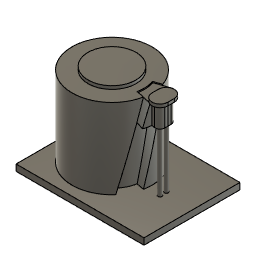
CAM+loft (Autodesk Fusion 360 design; units mm, degrees)
Autodesk Fusion 360 part; units mm, degrees
cylinder "CylinderPrimitive1" add diameter 25 height 25 placed x (1, 0, 0) y (0, 0, -1) z (0, 1, 0) at (0, 0, 0) makes body 1 in component "CAM"
ref_plane "WorkPlane1" through (0, 12.5, 0) normal (0, 1, 0) x (1, 0, 0)
ref_plane "WorkPlane2" through (0, 6.25, 0) normal (0, 1, 0) x (0, 0, 1)
ref_plane "WorkPlane3" through (0, 18.75, 0) normal (0, 1, 0) x (1, 0, 0)
sketch "Sketch2" plane through (0, 0, 0) normal (0, -1, 0) x (1, 0, 0)
  circle A0 centre (0, 0) radius 12.5
  line L0 (10, 0) -> (15, 0)
  line L1 (8.6603, 5) -> (12.9904, 7.5)
  arc A1 (15, 0) -> (12.9904, 7.5) centre (0, 0) ccw
  arc A2 (10, 0) -> (8.6603, 5) centre (0, 0) ccw
  line L2 (8.6603, 5) -> (0, 0) construction
  line L3 (0, 0) -> (10, 0) construction
  line L4 (0, 0) -> (14.4889, 3.8823) construction
  line L5 (9.6593, 2.5882) -> (14.4889, 3.8823) construction
  point P0 (12.0741, 3.2352)
  dimension "d3" = 30
  dimension "d4" = 30
  dimension "d5" = 20
  constraint horizontal L0
  constraint coincident A0.centre A1.centre
  constraint parallel L1 L2
  constraint parallel L0 L3
  constraint midpoint A1 L4.end
  constraint midpoint A2 L5.start
  constraint midpoint L5 P0
  measures "d3" diameter of A1
  measures "d4" angle of L0 L1
  measures "d5" diameter of A2
sketch "Sketch3" plane through (0, 6.25, 0) normal (0, 1, 0) x (1, 0, 0)
  circle A0 centre (0, 0) radius 12.5 construction
  line L0 (9.2388, -3.8268) -> (13.8582, -5.7403)
  line L1 (9.9144, 1.3053) -> (14.8717, 1.9579)
  line L2 (0, 0) -> (15, 0) construction
  line L3 (10, 0) -> (15, 0) construction
  arc A1 (9.2388, -3.8268) -> (9.9144, 1.3053) centre (0, 0) ccw
  arc A2 (13.8582, -5.7403) -> (14.8717, 1.9579) centre (0, 0) ccw
  line L4 (9.2388, -3.8268) -> (0, 0) construction
  line L5 (9.9144, 1.3053) -> (0, 0) construction
  line L6 (0, 0) -> (14.8717, -1.9579) construction
  line L7 (14.8717, -1.9579) -> (9.9144, -1.3053) construction
  point P0 (12.3931, -1.6316)
  dimension "d6" = 30
  dimension "d7" = 20
  dimension "d8" = 30
  dimension "d9" = 7.5
  constraint concentric A0 A2
  constraint concentric A0 A1
  constraint coincident A0.centre L2.start
  constraint coincident L2.end A2
  constraint horizontal L2
  constraint parallel L0 L4
  constraint midpoint A2 L6.end
  constraint midpoint A1 L7.end
  constraint parallel L6 L7
  constraint midpoint L7 P0
  measures "d6" diameter of A2
  measures "d7" diameter of A1
  measures "d8" angle of L0 L1
  measures "d9" angle of L1 L3
sketch "Sketch4" plane through (0, 12.5, 0) normal (0, 1, 0) x (1, 0, 0)
  line L0 (9.6593, -2.5882) -> (14.4889, -3.8823) construction
  line L1 (0, 0) -> (15, 0) construction
  line L2 (9.6593, 2.5882) -> (14.4889, 3.8823)
  line L3 (0, 0) -> (14.4889, -3.8823) construction
  line L4 (10, 0) -> (15, 0) construction
  arc A0 (9.6593, -2.5882) -> (9.6593, 2.5882) centre (0, 0) ccw
  arc A1 (14.4889, -3.8823) -> (14.4889, 3.8823) centre (0, 0) ccw
  line L5 (14.4889, -3.8823) -> (9.6593, -2.5882)
  line L6 (9.6593, 2.5882) -> (0, 0) construction
  point P0 (12.5, 0)
  dimension "d10" = 30
  dimension "d11" = 20
  dimension "d13" = 30
  dimension "d14" = 15
  dimension "d15" = 30
  constraint coincident L1.start L3.start
  constraint concentric A0 A1
  constraint coincident L1.end A1
  constraint horizontal L1
  constraint coincident L0.end L3.end
  constraint parallel L3 L5
  constraint midpoint L4 P0
  measures "d10" diameter of A1
  measures "d11" diameter of A0
  measures "d13" angle of L0 L2
  measures "d14" angle of L2 L4
  measures "d15" angle of L3 L6
sketch "Sketch5" plane through (0, 18.75, 0) normal (0, 1, 0) x (1, 0, 0)
  line L0 (0, 0) -> (13.8582, 5.7403)
  line L1 (10, 0) -> (15, 0) construction
  arc A0 (14.8717, -1.9579) -> (13.8582, 5.7403) centre (0, 0) ccw
  arc A1 (9.9144, -1.3053) -> (9.2388, 3.8268) centre (0, 0) ccw
  line L2 (14.8717, -1.9579) -> (9.9144, -1.3053)
  line L3 (9.9144, -1.3053) -> (0, 0) construction
  line L4 (9.9144, 1.3053) -> (14.8717, 1.9579) construction
  point P0 (12.3931, 1.6316)
  dimension "d16" = 30
  dimension "d17" = 20
  dimension "d20" = 30
  dimension "d21" = 7.5
  constraint coincident L0.start A0.centre
  constraint concentric A0 A1
  constraint coincident L0 A1.end
  constraint parallel L2 L3
  constraint midpoint A1 L4.start
  constraint midpoint A0 L4.end
  constraint midpoint L4 P0
  measures "d16" diameter of A0
  measures "d17" diameter of A1
  measures "d20" angle of L0 L2
  measures "d21" angle of L1 L2
sketch "Sketch6" plane through (0, 25, 0) normal (0, 1, 0) x (-1, 0, 0)
  circle A0 centre (0, 0) radius 12.5
  line L0 (-10, 0) -> (-15, 0)
  line L1 (-8.6603, -5) -> (-12.9904, -7.5)
  arc A1 (-15, 0) -> (-12.9904, -7.5) centre (0, 0) ccw
  arc A2 (-10, 0) -> (-8.6603, -5) centre (0, 0) ccw
  line L2 (-8.6603, -5) -> (0, 0) construction
  line L3 (-10, 0) -> (0, 0) construction
  line L4 (-9.6593, -2.5882) -> (-14.4889, -3.8823) construction
  point P0 (-12.0741, -3.2352)
  dimension "d22" = 30
  dimension "d23" = 20
  dimension "d24" = 30
  constraint coincident A0.centre A1.centre
  constraint horizontal L0
  constraint parallel L1 L2
  constraint parallel L0 L3
  constraint midpoint A2 L4.start
  constraint midpoint A1 L4.end
  constraint midpoint L4 P0
  measures "d22" diameter of A1
  measures "d23" diameter of A2
  measures "d24" angle of L0 L1
ref_plane "WorkPlane4" through (12.0741, 25, -3.2352) normal (0.56206, -0.178532, -0.807598) x (0.302733, 0.953075, 0)
ref_plane "WorkPlane5" through (12.3931, 18.75, -1.6316) normal (0.662664, -0.178532, -0.727326) x (0.260139, 0.965571, 0)
ref_plane "WorkPlane6" through (12.5, 12.5, 0) normal (0.75193, -0.178532, -0.634608) x (0.231009, 0.972952, 0)
ref_plane "WorkPlane7" through (12.0741, 0, 3.2352) normal (-0.82833, 0.178532, 0.531033) x (-0.210694, -0.977552, 0)
sketch "Sketch7" plane through (2.7742, -0.8812, -3.9862) normal (0.56206, -0.178532, -0.807598) x (0.302733, 0.953075, 0)
  line L0 (21.622, 3.9926) -> (27.4821, 1.2733)
  point P0 (21.622, 3.9926)
  point P1 (27.4821, 1.2733)
  constraint coincident P0 L0.start
  constraint coincident P1 L0.end
sketch "Sketch8" plane through (4.0102, -1.0804, -4.4015) normal (0.662664, -0.178532, -0.727326) x (0.260139, 0.965571, 0)
  line L0 (15.3214, 6.4135) -> (21.3284, 4.0361)
  point P0 (15.3214, 6.4135)
  point P1 (21.3284, 4.0361)
  constraint coincident P0 L0.start
  constraint coincident P1 L0.end
sketch "Sketch9" plane through (5.3894, -1.2796, -4.5485) normal (0.75193, -0.178532, -0.634608) x (0.231009, 0.972952, 0)
  line L0 (8.9439, 7.9967) -> (15.0495, 5.8855)
  point P0 (8.9439, 7.9967)
  point P1 (15.0495, 5.8855)
  constraint coincident P0 L0.start
  constraint coincident P1 L0.end
sketch "Sketch10" plane through (6.8613, -1.4788, -4.3987) normal (-0.82833, 0.178532, 0.531033) x (-0.210694, -0.977552, 0)
  line L0 (-2.5439, 9.0092) -> (-8.7208, 7.1166)
  point P0 (-2.5439, 9.0092)
  point P1 (-8.7208, 7.1166)
  constraint coincident P0 L0.start
  constraint coincident P1 L0.end
ref_plane "WorkPlane8" through (8.6603, 25, -5) normal (-0.477136, -0.298938, -0.826424) x (0.530928, -0.847417, 0)
ref_plane "WorkPlane9" through (9.2388, 18.75, -3.8268) normal (-0.365184, -0.298938, -0.881633) x (0.633429, -0.7738, 0)
ref_plane "WorkPlane10" through (9.6593, 12.5, -2.5882) normal (-0.246984, -0.298938, -0.921756) x (0.770917, -0.636935, 0)
ref_plane "WorkPlane11" through (9.9144, 6.25, -1.3053) normal (-0.124558, -0.298938, -0.946109) x (0.923077, -0.384615, 0)
sketch "Sketch11" plane through (3.5659, 2.2341, 6.1762) normal (-0.477136, -0.298938, -0.826424) x (0.530928, -0.847417, 0)
  line L0 (-8.5314, -21.1643) -> (-14.2885, -24.2897)
  point P0 (-14.2885, -24.2897)
  point P1 (-8.5314, -21.1643)
  constraint coincident P1 L0.start
  constraint coincident P0 L0.end
sketch "Sketch12" plane through (2.0469, 1.6756, 4.9416) normal (-0.365184, -0.298938, -0.881633) x (0.633429, -0.7738, 0)
  line L0 (-0.4948, -18.6973) -> (-5.7306, -22.6342)
  point P0 (-0.4948, -18.6973)
  point P1 (-5.7306, -22.6342)
  constraint coincident P0 L0.start
  constraint coincident P1 L0.end
sketch "Sketch13" plane through (0.9229, 1.1171, 3.4444) normal (-0.246984, -0.298938, -0.921756) x (0.770917, -0.636935, 0)
  line L0 (7.484, -13.9316) -> (3.208, -18.8943)
  point P0 (7.484, -13.9316)
  point P1 (3.208, -18.8943)
  constraint coincident P0 L0.start
  constraint coincident P1 L0.end
sketch "Sketch14" plane through (0.2327, 0.5585, 1.7677) normal (-0.124558, -0.298938, -0.946109) x (0.923077, -0.384615, 0)
  line L0 (13.8462, -5.4583) -> (11.3239, -11.504)
  point P0 (13.8462, -5.4583)
  point P1 (11.3239, -11.504)
  constraint coincident P0 L0.start
  constraint coincident P1 L0.end
loft "Loft1" cut profiles "Sketch6", "Sketch5", "Sketch4", "Sketch3", "Sketch2" section 1 contours A0 L0 L1 A2 | A0 L0 L1 A1 picked at (-10.5375, -4.9535) section 2 section 3 section 4 section 5 contours A0 L0 L1 A2 | A0 L0 L1 A1 picked at (10.5375, 4.9535) bodies 1 in component "CAM"
loft "Loft1'" add profiles "Sketch6", "Sketch5" section 1 contours A0 L0 L1 A2 | A0 L0 L1 A1 picked at (-10.5375, -4.9535) section 2 separate body makes body 2 in component "Driver"
sketch "Sketch1" plane through (0, 25, 0) normal (0, 1, 0) x (-1, 0, 0) in component "CAM"
  line L0 (-8.6603, -5) -> (-10.8253, -6.25)
  arc A0 (-10.8253, -6.25) -> (-12.5, 0) centre (0, 0) ccw
  line L1 (-12.5, 0) -> (-10, 0)
  spline S0 degree 3 poles (-10, 0) (-10, -1.7453) (-9.5329, -3.4885) (-8.6603, -5) knots -1 -1 -1 -1 0 0 0 0
  circle A1 centre (0, 0) radius 2.5
  dimension "d28" = 5
  constraint concentric A0 A1
  measures "d28" diameter of A1
extrude "Extrude1" cut sketch "Sketch1" against normal blind 25 contours A1 bodies 1 in component "CAM"
move_body "Move1" bodies 1 to x (0.965926, 0, 0.258819) y (0, 1, 0) z (-0.258819, 0, 0.965926) at (0, 0, 0) in component "CAM"
move_body "Move1'" bodies 2 to x (0.965926, 0, 0.258819) y (0, 1, 0) z (-0.258819, 0, 0.965926) at (0, 0, 0) in component "Driver"
sketch "Sketch15" plane through (0, 0, 0) normal (0, 1, 0) x (1, 0, 0)
  line L0 (-15, 15) -> (25, 15)
  line L1 (25, 15) -> (25, -15)
  line L2 (25, -15) -> (-15, -15)
  line L3 (-15, -15) -> (-15, 15)
  dimension "d31" = 40
  dimension "d32" = 30
  dimension "d33" = 15
  dimension "d34" = 25
  constraint horizontal L0
  constraint vertical L1
  constraint horizontal L2
  constraint vertical L3
  measures "d31" distance of L0.start L0.end
  measures "d32" distance of L0.start L2.end
  measures "d33" distance of origin L0
  measures "d34" distance of origin L1
extrude "Extrude1'" add sketch "Sketch15" against normal blind 2 separate body makes body 3 in component "Baseplate"
sketch "Sketch1 (2)" plane through (0, 0, 0) normal (0, 1, 0) x (-1, 0, 0) in component "Baseplate"
  line L0 (15, 15) -> (-25, 15)
  line L1 (-25, 15) -> (-25, -15)
  line L2 (-25, -15) -> (15, -15)
  line L3 (15, -15) -> (15, 15)
  circle A0 centre (0, 0) radius 2.25
  dimension "d37" = 4.5
  constraint coincident A0.centre origin
  measures "d37" diameter of A0
extrude "Extrude2" add sketch "Sketch1 (2)" along normal blind 25.5 contours A0 bodies 3 in component "Baseplate"
sketch "Sketch2 (2)" plane through (0, 25.5, 0) normal (0, 1, 0) x (-1, 0, 0) in component "Baseplate"
  circle A0 centre (0, 0) radius 2.25
  circle A1 centre (0, 0) radius 7.5
  dimension "d40" = 15
  constraint coincident A0.centre A1.centre
  measures "d40" diameter of A1
extrude "Extrude3" add sketch "Sketch2 (2)" along normal blind 1 contours A0 | A1 bodies 3 in component "Baseplate"
move_face "OffsetFaces1" offset -0.1 2 faces at (12.083, 19.4444, -1.7695) (11.8648, 19.4444, 4.714) on bodies 2 in component "Driver"
sketch "Sketch3 (2)" plane through (0, 0, 0) normal (0, 1, 0) x (-1, 0, 0) in component "Baseplate"
  circle A0 centre (0, 0) radius 2.25
  line L0 (15, 15) -> (-25, 15)
  line L1 (-25, 15) -> (-25, -15)
  line L2 (-25, -15) -> (15, -15)
  line L3 (15, -15) -> (15, 15)
  circle A1 centre (-16, -1) radius 0.625
  circle A2 centre (-16, 1) radius 0.625
  dimension "d44" = 1.25
  dimension "d45" = 1.25
  dimension "d46" = 2
  dimension "d47" = 1
  dimension "d48" = 16
  dimension "d49" = 16
  measures "d44" diameter of A1
  measures "d45" diameter of A2
  measures "d46" distance of A1.centre A2.centre
  measures "d47" vertical distance of A0.centre A1.centre
  measures "d48" horizontal distance of A0.centre A1.centre
  measures "d49" horizontal distance of A0.centre A2.centre
extrude "Extrude4" add sketch "Sketch3 (2)" along normal blind 25.5 contours A1 | A2 bodies 3 in component "Baseplate"
sketch "Sketch4 (2)" plane through (0, 25.5, 0) normal (0, 1, 0) x (-1, 0, 0) in component "Baseplate"
  circle A0 centre (-16, -1) radius 0.625
  circle A1 centre (-16, 1) radius 0.625 construction
  line L0 (-13.5, -1) -> (-13.5, 1)
  arc A2 (-13.5, 1) -> (-18.5, 1) centre (-16, 1) ccw
  line L1 (-18.5, 1) -> (-18.5, -1)
  arc A3 (-18.5, -1) -> (-13.5, -1) centre (-16, -1) ccw
  line L2 (-16, -1) -> (-16, 1) construction
  dimension "d52" = 5
  constraint tangent L0 A2
  constraint tangent A2 L1
  constraint parallel L0 L1
  constraint tangent L1 A3
  constraint tangent L0 A3
  constraint coincident A1.centre A2.centre
  constraint vertical L2
  constraint coincident A0.centre A3.centre
  measures "d52" diameter of A2
extrude "Extrude5" add sketch "Sketch4 (2)" along normal blind 1 contours A0 | L0 A2 L1 A3 bodies 3 in component "Baseplate"
sketch "Sketch1 (3)" plane through (0, 25, 0) normal (0, 1, 0) x (-1, 0, 0) in component "Driver"
  arc A0 (-14.5157, 3.781) -> (-14.5157, -3.781) centre (0, 0) ccw
  spline S0 degree 3 poles (-14.5157, -3.781) (-14.3218, -3.7291) (-14.1279, -3.6773) (-12.5154, -3.2463) (-11.1002, -2.8679) (-9.6852, -2.4894) knots 0.87539 0.87539 0.87539 0.87539 0.935572 0.935572 1.375809 1.375809 1.375809 1.375809
  arc A1 (-9.6852, 2.4894) -> (-9.6852, -2.4894) centre (0, 0) ccw
  spline S1 degree 3 poles (-9.6852, 2.4894) (-11.1004, 2.8679) (-12.5158, 3.2464) (-14.1283, 3.6774) (-14.322, 3.7292) (-14.5157, 3.781) knots 0.496573 0.496573 0.496573 0.496573 0.937318 0.937318 0.9975 0.9975 0.9975 0.9975
  circle A2 centre (-16, -1) radius 0.625 construction
  circle A3 centre (-16, -1) radius 0.625 construction
  circle A4 centre (-16, 1) radius 0.625 construction
  circle A5 centre (-16, 1) radius 0.625 construction
  circle A6 centre (-16, -1) radius 0.725
  circle A7 centre (-16, 1) radius 0.725
  line L0 (0, 0) -> (-9.9421, -1.0745) construction
  line L1 (-14.9132, -1.6118) -> (-15.9221, -1.7208)
  line L2 (0, 0) -> (-9.9421, 1.0745) construction
  line L3 (-14.9132, 1.6118) -> (-15.9221, 1.7208)
  line L4 (-16.0125, -0.2751) -> (-14.9978, -0.2577)
  line L5 (-9.9985, -0.1718) -> (0, 0) construction
  line L6 (0, 0) -> (-9.9985, 0.1718) construction
  line L7 (-14.9978, 0.2577) -> (-16.0125, 0.2751)
  line L8 (-15, 0) -> (0, 0) construction
  line L9 (-15, 0) -> (-17.5, 0) construction
  line L10 (-17.5, 0) -> (-17.5, 1)
  arc A8 (-16.4494, -0.4311) -> (-16.3229, -0.4648) centre (-16, 1) ccw construction
  arc A9 (-15.7668, 2.4818) -> (-17.5, 1) centre (-16, 1) ccw
  line L11 (0, 0) -> (-9.8784, 1.5549) construction
  line L12 (-14.8176, 2.3323) -> (-15.7668, 2.4818)
  line L13 (-14.8176, -2.3323) -> (-15.7668, -2.4818)
  arc A10 (-17.5, -1) -> (-15.7668, -2.4818) centre (-16, -1) ccw
  line L14 (-17.5, 0) -> (-17.5, -1)
  dimension "d55" = 0.1
  dimension "d56" = 0.1
  dimension "d57" = 2.5
  dimension "d58" = 1.5
  dimension "d59" = 1
  constraint coincident A0.centre A1.centre
  constraint coincident A6 L1.end
  constraint tangent A6 L0
  constraint coincident A7 L3.end
  constraint coincident A1 L0.end
  constraint coincident A0 L1.start
  constraint collinear L0 L1
  constraint coincident A1 L2.end
  constraint coincident A0 L3.start
  constraint collinear L2 L3
  constraint coincident A6 L4.start
  constraint coincident A7 L7.end
  constraint tangent A7 L6
  constraint tangent A6 L4
  constraint coincident A0 L4.end
  constraint coincident A1 L5.start
  constraint collinear L4 L5
  constraint coincident A1 L6.end
  constraint coincident A0 L7.start
  constraint collinear L6 L7
  constraint tangent A7 L3
  constraint midpoint A0 L8.start
  constraint parallel L8 L9
  constraint concentric A4 A8
  constraint coincident A9.start A8
  constraint tangent A8 L11
  constraint tangent L10 A8
  constraint vertical L10
  constraint coincident A6 A8.start
  constraint coincident A2 A8.end
  constraint coincident A1 L11.end
  constraint coincident A0 L12.start
  constraint collinear L11 L12
  constraint symmetric A9.start L8 L13.end
  constraint symmetric L8 L9.end L10.start
  constraint symmetric L8 L10.end A10.start
  constraint symmetric L8 A9 A10
  constraint symmetric L8 L12.start L13.start
  measures "d57" distance of L8.start L9.end
  measures "d58" radius of A9
  measures "d59" distance of L9.end L10.end
move_body "Move2" bodies 1 to x (0.997859, 0, -0.065403) y (0, 1, 0) z (0.065403, 0, 0.997859) at (0, 0, 0) in component "CAM"
move_body "Move2'" bodies 2 to x (0.997859, 0, -0.065403) y (0, 1, 0) z (0.065403, 0, 0.997859) at (0, 0, 0) in component "Driver"
extrude "Extrude1''" add sketch "Sketch1 (3)" against normal blind 6.25 contours A0 A6 A7 L1 L3 L4 L7 L10 A9 L12 L13 A10 L14 bodies 2 in component "Driver"
move_face "OffsetFaces2" offset -0.1 1 faces at (9.7731, 22.2222, -2.0114) on bodies 2 in component "Driver"
component "CAM" placed x (1, 0, 0) y (0, 1, 0) z (0, 0, 1) at (0, 0.2456, 0)
component "Driver" placed x (1, 0, 0) y (0, 1, 0) z (0, 0, 1) at (0, 0, 0)
component "Baseplate" placed x (1, 0, 0) y (0, 1, 0) z (0, 0, 1) at (0, -0.25, 0)
